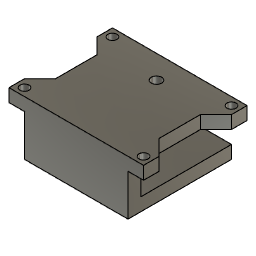
Pulley Bracket (Autodesk Fusion 360 design; units mm, degrees)
Autodesk Fusion 360 part; units mm, degrees
sketch "Sketch1" plane through (0, 0, 0) normal (1, 0, 0) x (0, 1, 0) in component "ㄷ bracket v12"
  line L0 (0, 21) -> (40, 21)
  line L1 (40, 21) -> (40, 16)
  line L2 (0, 40.0001) -> (0, 21)
  line L3 (0, 40.0001) -> (0, 0)
  line L4 (0, 0) -> (40, 0)
  line L5 (5, 16) -> (5, 5)
  line L6 (5, 5) -> (40, 5)
  line L7 (40, 0) -> (40, 5)
  line L8 (5, 16) -> (40, 16)
  dimension "d6" = 5
  dimension "d7" = 5
  dimension "d8" = 40
  dimension "d9" = 21
  constraint horizontal L0
  constraint vertical L1
  constraint vertical L2
  constraint perpendicular L3 L4
  constraint perpendicular L5 L6
  constraint perpendicular L6 L7
  constraint perpendicular L1 L8
  constraint parallel L1 L7
  constraint equal L1 L7
  constraint equal L0 L4
  constraint coincident L3.end L4.start
  measures "d6" distance of L0 L8
  measures "d7" distance of L3 L5
  measures "d8" distance of L0.start L0.end
  measures "d9" distance of L0 L4
extrude "Extrude1" add sketch "Sketch1" along normal blind 40 in component "ㄷ bracket v12"
sketch "Sketch2" plane through (0, 0, 21) normal (0, 0, 1) x (-1, 0, 0) in component "ㄷ bracket v12"
  line L0 (0, -40) -> (0, 0)
  line L1 (0, 0) -> (-40, 0)
  line L2 (-40, 0) -> (-40, -40)
  line L3 (-40, -40) -> (0, -40)
  circle A0 centre (-20, -31) radius 2
  line L4 (6, -40) -> (0, -40)
  line L5 (0, -40) -> (0, -34)
  line L6 (6, -34) -> (6, -40)
  line L7 (-40, -40) -> (-46, -40)
  line L8 (-46, -40) -> (-46, -34)
  line L9 (-40, -34) -> (-40, -40)
  line L10 (0, -6) -> (0, 0)
  line L11 (0, 0) -> (6, 0)
  line L12 (6, 0) -> (6, -6)
  line L13 (-46, -6) -> (-46, 0)
  line L14 (-46, 0) -> (-40, 0)
  line L15 (-40, 0) -> (-40, -6)
  circle A1 centre (3, -37) radius 1.75
  circle A2 centre (3, -3) radius 1.75
  circle A3 centre (-43, -3) radius 1.75
  circle A4 centre (-43, -37) radius 1.75
  line L16 (6, -34) -> (0, -28)
  line L17 (6, -34) -> (11.6569, -34) construction
  line L18 (0, -12) -> (0, -6)
  line L19 (0, -28) -> (0, -34)
  line L20 (6, -6) -> (0, -12)
  line L21 (-46, -6) -> (-40, -12)
  line L22 (-46, -6) -> (-37.5147, -6) construction
  line L23 (-40, -12) -> (-40, -6)
  line L24 (-46, -34) -> (-40, -28)
  line L25 (-40, -34) -> (-40, -28)
  dimension "d16" = 4
  dimension "d20" = 6
  dimension "d21" = 6
  dimension "d22" = 6
  dimension "d23" = 6
  dimension "d24" = 6
  dimension "d25" = 6
  dimension "d26" = 6
  dimension "d27" = 6
  dimension "d29" = 3.5
  dimension "d30" = 3
  dimension "d31" = 3
  dimension "d32" = 3.5
  dimension "d33" = 3.5
  dimension "d35" = 3
  dimension "d37" = 3
  dimension "d38" = 3.5
  dimension "d39" = 3
  dimension "d40" = 3
  dimension "d43" = 135
  dimension "d45" = 45
  dimension "d46" = 135
  dimension "d47" = 135
  dimension "d48" = 8.4853
  constraint horizontal L4
  constraint vertical L5
  constraint vertical L6
  constraint coincident L0 L5.end
  constraint horizontal L7
  constraint vertical L8
  constraint vertical L9
  constraint vertical L10
  constraint horizontal L11
  constraint vertical L12
  constraint coincident L0.end L1.start
  constraint vertical L13
  constraint horizontal L14
  constraint vertical L15
  constraint coincident L2 L15.end
  constraint coincident L1.end L2.start
  constraint coincident L0.start L3.end
  constraint coincident L2.end L3.start
  constraint horizontal L17
  constraint coincident L0 L16.end
  constraint horizontal L22
  constraint coincident L2 L21.end
  constraint coincident L2 L24.end
  measures "d16" diameter of A0
  measures "d20" distance of L0.start L4.start
  measures "d21" distance of L4.start L6.start
  measures "d22" distance of L12.end L10.start
  measures "d23" distance of L12.end L11.end
  measures "d24" distance of L2.end L7.end
  measures "d25" distance of L7.end L8.end
  measures "d26" distance of L15.end L13.start
  measures "d27" distance of L13.start L13.end
  measures "d29" diameter of A1
  measures "d30" distance of L4 A1.centre
  measures "d31" distance of L6 A1.centre
  measures "d32" diameter of A2
  measures "d33" diameter of A3
  measures "d35" distance of L12 A2.centre
  measures "d37" distance of L13 A3.centre
  measures "d38" diameter of A4
  measures "d39" distance of L7 A4.centre
  measures "d40" distance of L8 A4.centre
  measures "d43" angle of L16 L17
  measures "d45" angle of L21 L22
  measures "d46" angle of L23 L24
  measures "d47" angle of L12 L20
  measures "d48" distance of L12.end L18.start
hole "Hole1" at (21.8353, 19.3113, 21) direction (0, 0, -1) diameter 30 depth 125 tip angle 118 in component "ㄷ bracket v12"
move_face "OffsetFaces1" offset 5 2 faces at (18.8386, 4.6137, 8.6667) (18.8386, 4.6137, 8.6667) in component "ㄷ bracket v12"
move_face "OffsetFaces2" offset 3 2 faces at (22.831, 9.3609, 17.6667) (22.831, 9.3609, 3.3333) in component "ㄷ bracket v12"
move_face "OffsetFaces3" offset 3 2 faces at (22.5323, 12.346, 17.6667) (22.5323, 12.346, 3.3333) in component "ㄷ bracket v12"
move_face "OffsetFaces4" offset 2 2 faces at (22.2336, 15.3311, 17.6667) (22.2336, 15.3311, 3.3333) in component "ㄷ bracket v12"
move_face "OffsetFaces5" offset 5 1 faces at (22.0344, 17.3212, 17.6667) in component "ㄷ bracket v12"
move_face "OffsetFaces6" offset 5 1 faces at (22.0344, 17.3212, 3.3333) in component "ㄷ bracket v12"
hole "Hole2" at (20, 31, 21) direction (0, 0, -1) diameter 4 depth 30 tip angle 118 in component "ㄷ bracket v12"
extrude "Extrude2" add sketch "Sketch2" against normal blind 5 contours L0 L4 L5 L6 L16 L19 | L2 L7 L8 L9 L24 L25 | L0 L10 L11 L12 L18 L20 | L2 L13 L14 L15 L21 L23 in component "ㄷ bracket v12"
component "ㄷ bracket v12" placed x (1, 0, 0) y (0, 1, 0) z (0, 0, 1) at (0, 0, 0)
equation "d21 = d20"
equation "d22 = d20"
equation "d23 = d20"
equation "d24 = d20"
equation "d25 = d20"
equation "d26 = d20"
equation "d27 = d20"
equation "d30 = d20 / 2"
equation "d31 = d30"
equation "d32 = d29"
equation "d33 = d29"
equation "d35 = d30"
equation "d37 = d30"
equation "d38 = d29"
equation "d39 = d30"
equation "d40 = d30"
